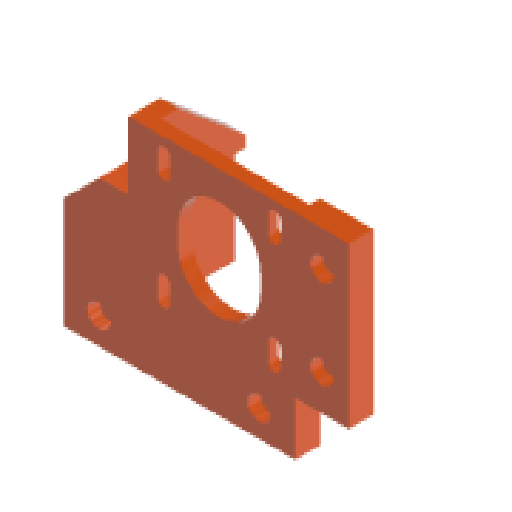
# Autodesk Inventor part: Alpha Motor Mount
Saved by Autodesk Inventor 2023.2 (Build 272271000, 271)
## iProperties
Created: 2023-02-03
Part Number: Alpha Motor Mount
Material: ABS Plastic
Document SubType Name: Modeling
Designer: remop
Density: 1.06 g/cm^3
Appearance: Smooth - Light Orange
Author: remop
Autodesk Inventor part; units mm, degrees
ref_plane "YZ Plane" through (0, 0, 0) normal (1, 0, 0) x (0, 1, 0)
ref_plane "XZ Plane" through (0, 0, 0) normal (0, 1, 0) x (-1, 0, 0)
ref_plane "XY Plane" through (0, 0, 0) normal (0, 0, 1) x (1, 0, 0)
sketch "Sketch1" plane through (0, 0, 0) normal (0, 0, 1) x (1, 0, 0)
  line L0 (0, 0) -> (0, 15)
  line L1 (0, 15) -> (15, 15)
  line L2 (15, 15) -> (15, 60)
  line L3 (15, 60) -> (-65, 60)
  line L4 (-65, 60) -> (-65, 0)
  line L5 (-65, 0) -> (0, 0)
  line L6 (-36.8, 25) -> (-36.8, 20) construction
  line L7 (-38.4, 25) -> (-38.4, 20)
  line L8 (-35.2, 20) -> (-35.2, 25)
  arc A0 (-35.2, 25) -> (-38.4, 25) centre (-36.8, 25) ccw
  arc A1 (-38.4, 20) -> (-35.2, 20) centre (-36.8, 20) ccw
  line L9 (-5.8, 25) -> (-5.8, 20) construction
  line L10 (-7.4, 25) -> (-7.4, 20)
  line L11 (-4.2, 20) -> (-4.2, 25)
  arc A2 (-4.2, 25) -> (-7.4, 25) centre (-5.8, 25) ccw
  arc A3 (-7.4, 20) -> (-4.2, 20) centre (-5.8, 20) ccw
  line L12 (-5.8, 56) -> (-5.8, 51) construction
  line L13 (-7.4, 56) -> (-7.4, 51)
  line L14 (-4.2, 51) -> (-4.2, 56)
  arc A4 (-4.2, 56) -> (-7.4, 56) centre (-5.8, 56) ccw
  arc A5 (-7.4, 51) -> (-4.2, 51) centre (-5.8, 51) ccw
  line L15 (-36.8, 56) -> (-36.8, 51) construction
  line L16 (-38.4, 56) -> (-38.4, 51)
  line L17 (-35.2, 51) -> (-35.2, 56)
  arc A6 (-35.2, 56) -> (-38.4, 56) centre (-36.8, 56) ccw
  arc A7 (-38.4, 51) -> (-35.2, 51) centre (-36.8, 51) ccw
  line L18 (-21.3, 40.5) -> (-21.3, 35.5) construction
  line L19 (-32.8, 40.5) -> (-32.8, 35.5)
  line L20 (-9.8, 35.5) -> (-9.8, 40.5)
  arc A8 (-9.8, 40.5) -> (-32.8, 40.5) centre (-21.3, 40.5) ccw
  arc A9 (-32.8, 35.5) -> (-9.8, 35.5) centre (-21.3, 35.5) ccw
  line L21 (-41.8, 60) -> (-41.8, 41)
  line L22 (-41.8, 41) -> (-55, 41)
  line L23 (-55, 41) -> (-65, 31)
  point P0 (-36.8, 22.5)
  point P1 (-5.8, 22.5)
  point P2 (-5.8, 53.5)
  point P3 (-36.8, 53.5)
  point P4 (-21.3, 38)
  dimension "d0" = 15
  dimension "d57" = 3.2
  dimension "d58" = 31
  dimension "d59" = 31
  dimension "d60" = 36.3
  dimension "d61" = 11.5
  dimension "d62" = 5
  dimension "d63" = 15.5
  dimension "d64" = 15.5
  dimension "d65" = 60
  dimension "d66" = 80
  dimension "d67" = 38
  dimension "d68" = 45
  dimension "d69" = 31
  dimension "d70" = 19
  dimension "d71" = 5
  constraints: 58 end point, 20 point on circle, 20 tangent, 10 centre point, 7 parallel, 6 perpendicular, 5 equal length, 5 midpoint, 4 point on line, 4 vertical, 3 equal radius, 2 horizontal alignment, 2 vertical alignment
  measures "d0" distance of L0.start L0.end
  measures "d57" distance between parallel lines of L8 L7
  measures "d58" distance of point (-5.8, 22.5) point (-36.8, 22.5)
  measures "d59" distance of point (-36.8, 53.5) point (-36.8, 22.5)
  measures "d60" distance from line of L2 point (-21.3, 38)
  measures "d61" radius of A9
  measures "d62" distance of L19.start L19.end
  measures "d63" distance from line of L18 point (-36.8, 22.5)
  measures "d64" horizontal distance of point (-36.8, 22.5) point (-21.3, 38)
  measures "d65" distance of L3.end L4.end
  measures "d66" distance of L2.end L3.end
  measures "d67" distance from line of L5 point (-21.3, 38)
  measures "d68" angle of L4 L23
  measures "d69" distance from line of L5 L23.end
  measures "d70" distance of L21.start L21.end
  measures "d71" distance from line of point (-36.8, 53.5) L21
extrude "Extrusion1" add sketch "Sketch1" along normal blind 4 contours L5 L4 L23 L22 L21 L3 L2 L1 L0
sketch "Sketch2" plane through (0, 0, 0) normal (0, 0, -1) x (-1, 0, 0)
  line L0 (0, 15) -> (-15, 15) projected
  line L1 (0, 0) -> (0, 15) projected
  line L2 (65, 0) -> (0, 0) projected
  line L3 (65, 31) -> (65, 0) projected
  line L4 (-15, 60) -> (41.8, 60) projected
  line L5 (-15, 15) -> (-15, 60) projected
  line L6 (0, 15) -> (65, 15)
  line L7 (65, 31) -> (65, 0) projected
  line L8 (0, 15) -> (-15, 15) projected
  line L9 (0, 15) -> (0, 60)
  line L10 (-15, 60) -> (41.8, 60) projected
  line L11 (55, 41) -> (65, 31) projected
  line L12 (41.8, 41) -> (55, 41) projected
  line L13 (41.8, 60) -> (41.8, 41) projected
  point P0 (65, 60)
  point P1 (0, 60)
  constraints: 4 end point, 2 perpendicular, 2 point on line
extrude "Extrusion2" add sketch "Sketch2" along normal blind 3 contours L6 L3 L2 L1 | L0 L5 L4 L9
sketch "Sketch3" plane through (0, 0, 4) normal (0, 0, 1) x (1, 0, 0)
  line L0 (-65, 31) -> (-65, 0) projected
  line L1 (-65, 0) -> (0, 0) projected
  line L2 (0, 0) -> (0, 15) projected
  line L3 (0, 15) -> (15, 15) projected
  line L4 (15, 15) -> (15, 60) projected
  line L5 (15, 60) -> (-41.8, 60) projected
  line L6 (-65, 0) -> (-65, 15) projected
  line L7 (0, 60) -> (15, 60) projected
  line L8 (-41.8, 60) -> (-41.8, 41) projected
  line L9 (-41.8, 41) -> (-55, 41) projected
  line L10 (-55, 41) -> (-65, 31) projected
  point P0 (-10, 7.5)
  point P1 (-55, 7.5)
  point P2 (7.5, 25)
  point P3 (7.5, 50)
  point P4 (0, 7.5)
  point P5 (-65, 7.5)
  point P6 (7.5, 15)
  point P7 (7.5, 60)
  dimension "d18" = 10
  dimension "d19" = 10
  dimension "d20" = 10
  dimension "d21" = 10
  constraints: 4 midpoint, 2 horizontal alignment, 2 vertical alignment
  measures "d18" distance from line of L2 point (-10, 7.5)
  measures "d19" distance from line of L6 point (-55, 7.5)
  measures "d20" distance from line of L3 point (7.5, 25)
  measures "d21" distance from line of L7 point (7.5, 50)
hole "Hole1" at (-10, 7.5, 4) at (-55, 7.5, 4) at (7.5, 25, 4) at (7.5, 50, 4) direction (0, 0, -1) diameter 3.6 end through all counterbore diameter 6.5 counterbore depth 3.4 clearance for "Socket Head Cap Screw ISO 4762" size "M3" standard "ISO"
sketch "Sketch8" plane through (0, 0, 0) normal (0, 0, -1) x (-1, 0, 0)
  line L0 (0, 15) -> (65, 15) projected
  line L1 (65, 31) -> (65, 15) projected
  line L2 (55, 41) -> (65, 31) projected
  line L3 (41.8, 41) -> (55, 41) projected
  line L4 (41.8, 60) -> (41.8, 41) projected
  line L5 (0, 60) -> (41.8, 60) projected
  line L6 (0, 60) -> (0, 15) projected
  arc A0 (32.8, 40.5) -> (9.8, 40.5) centre (21.3, 40.5) ccw projected
  line L7 (32.8, 35.5) -> (32.8, 40.5) projected
  arc A1 (9.8, 35.5) -> (32.8, 35.5) centre (21.3, 35.5) ccw projected
  line L8 (9.8, 40.5) -> (9.8, 35.5) projected
  arc A2 (38.4, 56) -> (35.2, 56) centre (36.8, 56) ccw projected
  line L9 (38.4, 51) -> (38.4, 56) projected
  arc A3 (35.2, 51) -> (38.4, 51) centre (36.8, 51) ccw projected
  line L10 (35.2, 56) -> (35.2, 51) projected
  arc A4 (7.4, 56) -> (4.2, 56) centre (5.8, 56) ccw projected
  line L11 (7.4, 51) -> (7.4, 56) projected
  arc A5 (4.2, 51) -> (7.4, 51) centre (5.8, 51) ccw projected
  line L12 (4.2, 56) -> (4.2, 51) projected
  arc A6 (7.4, 25) -> (4.2, 25) centre (5.8, 25) ccw projected
  line L13 (7.4, 20) -> (7.4, 25) projected
  arc A7 (4.2, 20) -> (7.4, 20) centre (5.8, 20) ccw projected
  line L14 (4.2, 25) -> (4.2, 20) projected
  arc A8 (38.4, 25) -> (35.2, 25) centre (36.8, 25) ccw projected
  line L15 (38.4, 20) -> (38.4, 25) projected
  arc A9 (35.2, 20) -> (38.4, 20) centre (36.8, 20) ccw projected
  line L16 (35.2, 25) -> (35.2, 20) projected
  line L17 (41.8, 41) -> (55, 41) projected
  line L18 (41.8, 41) -> (41.8, 15)
  point P0 (0, 0)
  constraints: 2 end point, 1 perpendicular, 1 point on line
extrude "Extrusion5" add sketch "Sketch8" along normal blind 21 contours L18 L3 L2 L1 L0
sketch "Sketch9" plane through (-41.8, 41, 4) normal (-1, 0, 0) x (0, 0, 1)
  line L0 (-4, 19) -> (-4, 0) projected
  line L1 (-4, 0) -> (0, 0) projected
  line L2 (0, 19) -> (0, 0) projected
  line L3 (-4, 19) -> (0, 19) projected
  line L4 (-4, 0) -> (0, 0) projected
  line L5 (-4, 0) -> (-28, 0)
  line L6 (-28, 0) -> (-28, 3)
  line L7 (-28, 3) -> (-9, 19)
  line L8 (-9, 19) -> (-4, 19)
  line L9 (0, 19) -> (-7, 19) projected
  line L10 (-21.4252, 2) -> (-7, 14.1475)
  line L11 (-7, 14.1475) -> (-7, 2)
  line L12 (-7, 2) -> (-21.4252, 2)
  point P0 (-4, -41)
  dimension "d74" = 24
  dimension "d75" = 3
  dimension "d76" = 5
  dimension "d77" = 5
  dimension "d78" = 3
  dimension "d79" = 2
  constraints: 14 end point, 2 horizontal, 2 vertical, 1 collinear, 1 parallel
  measures "d74" distance of L0.end L5.end
  measures "d75" distance of L5.end L6.end
  measures "d76" distance of L7.end L0.start
  measures "d77" distance between parallel lines of L7 L10
  measures "d78" distance between parallel lines of L0 L11
  measures "d79" distance between parallel lines of L1 L12
extrude "Extrusion6" add sketch "Sketch9" along normal blind 5
sketch "Sketch10" plane through (0, 0, 0) normal (0, 0, -1) x (-1, 0, 0)
  line L0 (41.8, 60) -> (41.8, 15) projected
  line L1 (0, 60) -> (41.8, 60) projected
  line L2 (0, 60) -> (0, 15) projected
  line L3 (0, 15) -> (41.8, 15) projected
  arc A0 (32.8, 40.5) -> (9.8, 40.5) centre (21.3, 40.5) ccw projected
  line L4 (32.8, 35.5) -> (32.8, 40.5) projected
  arc A1 (9.8, 35.5) -> (32.8, 35.5) centre (21.3, 35.5) ccw projected
  line L5 (9.8, 40.5) -> (9.8, 35.5) projected
  arc A2 (38.4, 56) -> (35.2, 56) centre (36.8, 56) ccw projected
  line L6 (38.4, 51) -> (38.4, 56) projected
  arc A3 (35.2, 51) -> (38.4, 51) centre (36.8, 51) ccw projected
  line L7 (35.2, 56) -> (35.2, 51) projected
  arc A4 (7.4, 56) -> (4.2, 56) centre (5.8, 56) ccw projected
  line L8 (7.4, 51) -> (7.4, 56) projected
  arc A5 (4.2, 51) -> (7.4, 51) centre (5.8, 51) ccw projected
  line L9 (4.2, 56) -> (4.2, 51) projected
  arc A6 (7.4, 25) -> (4.2, 25) centre (5.8, 25) ccw projected
  line L10 (7.4, 20) -> (7.4, 25) projected
  arc A7 (4.2, 20) -> (7.4, 20) centre (5.8, 20) ccw projected
  line L11 (4.2, 25) -> (4.2, 20) projected
  arc A8 (38.4, 25) -> (35.2, 25) centre (36.8, 25) ccw projected
  line L12 (38.4, 20) -> (38.4, 25) projected
  arc A9 (35.2, 20) -> (38.4, 20) centre (36.8, 20) ccw projected
  line L13 (35.2, 25) -> (35.2, 20) projected
  line L14 (36.8, 56) -> (36.8, 51) construction
  line L15 (40.05, 56) -> (40.05, 51)
  line L16 (33.55, 51) -> (33.55, 56)
  arc A10 (40.05, 56) -> (33.55, 56) centre (36.8, 56) ccw
  arc A11 (33.55, 51) -> (40.05, 51) centre (36.8, 51) ccw
  line L17 (5.8, 51) -> (5.8, 56) construction
  line L18 (2.55, 51) -> (2.55, 56)
  line L19 (9.05, 56) -> (9.05, 51)
  arc A12 (2.55, 51) -> (9.05, 51) centre (5.8, 51) ccw
  arc A13 (9.05, 56) -> (2.55, 56) centre (5.8, 56) ccw
  line L20 (5.8, 20) -> (5.8, 25) construction
  line L21 (2.55, 20) -> (2.55, 25)
  line L22 (9.05, 25) -> (9.05, 20)
  arc A14 (2.55, 20) -> (9.05, 20) centre (5.8, 20) ccw
  arc A15 (9.05, 25) -> (2.55, 25) centre (5.8, 25) ccw
  line L23 (36.8, 20) -> (36.8, 25) construction
  line L24 (40.05, 20) -> (40.05, 25)
  line L25 (33.55, 25) -> (33.55, 20)
  arc A16 (33.55, 20) -> (40.05, 20) centre (36.8, 20) ccw
  arc A17 (40.05, 25) -> (33.55, 25) centre (36.8, 25) ccw
  point P0 (0, 0)
  point P1 (36.8, 53.5)
  point P2 (5.8, 53.5)
  point P3 (5.8, 22.5)
  point P4 (36.8, 22.5)
  dimension "d82" = 6.5
  constraints: 32 end point, 16 point on circle, 16 tangent, 8 centre point, 7 parallel, 4 midpoint, 3 equal radius, 1 vertical
  measures "d82" distance between parallel lines of L25 L24
extrude "Extrusion7" cut sketch "Sketch10" against normal blind 1.5 contours L15 A11 L16 A10 | L18 A13 L19 A12 | L21 A15 L22 A14 | A16 L25 A17 L24
equation "\"d59\" = d58"
equation "\"d63\" = 0.5 * d58"
equation "\"d64\" = 0.5 * d59"
equation "\"d19\" = d18"
equation "\"d20\" = d18"
equation "\"d21\" = d20"
body "Solid1"
